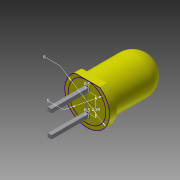
# Autodesk Inventor part: LED
Saved by Autodesk Inventor 2015 (Build 190159000, 159)
## iProperties
Created: 2015-06-12
Part Number: LED
Material: Generic
Document SubType Name: Modeling
Designer: Openlab
Density: 1 g/cm^3
Appearance: Default
Author: Openlab
Autodesk Inventor part; units mm, degrees
ref_plane "YZ Plane" through (0, 0, 0) normal (1, 0, 0) x (0, 1, 0)
ref_plane "XZ Plane" through (0, 0, 0) normal (0, 1, 0) x (-1, 0, 0)
ref_plane "XY Plane" through (0, 0, 0) normal (0, 0, 1) x (1, 0, 0)
sketch "Sketch1" plane through (0, 0, 0) normal (0, 1, 0) x (-1, 0, 0)
  arc A0 (-1.6583, 2.5) -> (1.6583, 2.5) centre (0, 0) ccw
  circle A1 centre (0, 0) radius 2.5
  line L0 (0.25, 1.77) -> (-0.25, 1.77)
  line L1 (-0.25, 1.77) -> (-0.25, 1.27)
  line L2 (-0.25, 1.27) -> (0.25, 1.27)
  line L3 (0.25, 1.27) -> (0.25, 1.77)
  line L4 (0, 1.87) -> (0, -2) construction
  line L5 (1.5109, 0) -> (-1.3865, 0) construction
  line L6 (0.25, -1.27) -> (-0.25, -1.27)
  line L7 (-0.25, -1.27) -> (-0.25, -1.77)
  line L8 (-0.25, -1.77) -> (0.25, -1.77)
  line L9 (0.25, -1.77) -> (0.25, -1.27)
  line L10 (-1.6583, 2.5) -> (1.6583, 2.5)
  dimension "d0" = 6
  dimension "d1" = 5
  dimension "d2" = 0.5
  dimension "d4" = 0.5
  dimension "d5" = 2.54
  constraints: 22 end point, 4 horizontal, 4 parallel, 4 perpendicular, 2 centre point, 2 coincident, 2 point on circle, 2 point on line, 1 tangent, 3 other
  measures "d0" diameter of A0
  measures "d1" diameter of A1
  measures "d2" distance of L2.end L1.end
  measures "d4" distance of L8.end L7.end
  measures "d5" distance between parallel lines of L6 L2
extrude "Extrusion1" add sketch "Sketch1" along normal blind 8.6 contours A1 | L3 L2 L1 L0 | L9 L8 L7 L6
extrude "Extrusion3" add sketch "Sketch1" along normal blind 1 contours L10 A0
fillet "Fillet1" radius 2.5 1 edges at (2.5, 8.6, 0)
extrude "Extrusion4" add sketch "Sketch1" against normal blind 5 contours L3 L2 L1 L0 | L9 L8 L7 L6
body "Solid1"
